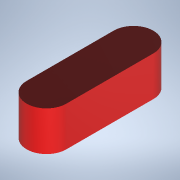
# Autodesk Inventor part: Passfeder12x5x5
Saved by Autodesk Inventor 2022 (Build 260153000, 153)
## iProperties
Created: 2022-03-11
Part Number: Passfeder12x5x5
Material: Generisch
Document SubType Name: Modeling
Designer: 123St
Density: 1 g/cm^3
Appearance: Rot
Mass: 0.223175 g
Surface Area: 2.1781 cm^2
Volume: 0.223175 cm^3
Passfeder_length: 16,000 mm
Passfeder_height: 6,000 mm
Passfeder_width: 6,000 mm
Wellennuttiefe: 3,500 mm
Nabennuttiefe: 2,800 mm
Author: 123St
Autodesk Inventor part; units mm, degrees
ref_plane "YZ Plane" through (0, 0, 0) normal (1, 0, 0) x (0, 1, 0)
ref_plane "XZ Plane" through (0, 0, 0) normal (0, 1, 0) x (-1, 0, 0)
ref_plane "XY Plane" through (0, 0, 0) normal (0, 0, 1) x (1, 0, 0)
sketch "Skizze1" plane through (0, 0, 0) normal (0, 1, 0) x (-1, 0, 0)
  line L0 (0, 5) -> (0, -5) construction
  line L1 (-3, 5) -> (-3, -5)
  line L2 (3, -5) -> (3, 5)
  arc A0 (3, 5) -> (-3, 5) centre (0, 5) ccw
  arc A1 (-3, -5) -> (3, -5) centre (0, -5) ccw
  line L3 (0, -11.2) -> (0, 11.2) construction
  point P0 (0, 0)
  point P1 (0, 0)
  point P2 (0, 8)
  point P3 (0, -8)
  dimension "d1" = 6
  dimension "d4" = 16
  constraints: 8 end point, 6 point on circle, 4 tangent, 2 centre point, 2 point on line, 1 coincident, 1 collinear, 1 midpoint, 1 parallel, 1 vertical
  measures "d1" distance between parallel lines of L1 L2
  measures "d4" distance of point (0, -8) point (0, 8)
extrude "Extrusion1" add sketch "Skizze1" along normal blind 6
equation "\"d1\" = Passfeder_width"
equation "\"d4\" = Passfeder_length"
equation "\"d2\" = Passfeder_height"
equation "\"Passfeder_height\" = 6"
equation "\"Passfeder_width\" = 6"
equation "\"Passfeder_length\" = 16"
equation "\"Wellennuttiefe\" = 3.5"
equation "\"Nabennuttiefe\" = 2.8"
